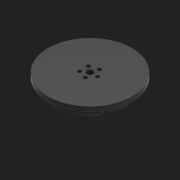
# Autodesk Inventor part: SE02
Saved by Autodesk Inventor 2017 (Build 210142000, 142)
## iProperties
Created: 2019-09-07
Part Number: SE02
Material: ABS Plastic
Document SubType Name: Modeling
Designer: Dell
Density: 1.06 g/cm^3
Appearance: Smooth - Black
Author: Dell
Autodesk Inventor part; units mm, degrees
ref_plane "YZ Plane" through (0, 0, 0) normal (1, 0, 0) x (0, 1, 0)
ref_plane "XZ Plane" through (0, 0, 0) normal (0, 1, 0) x (-1, 0, 0)
ref_plane "XY Plane" through (0, 0, 0) normal (0, 0, 1) x (1, 0, 0)
sketch "Sketch1" plane through (0, 0, 0) normal (0, 0, 1) x (1, 0, 0)
  circle A0 centre (0, 0) radius 15
  circle A1 centre (0, 0) radius 3.5
  dimension "d0" = 30
  dimension "d1" = 7
  constraints: 2 centre point, 2 coincident
  measures "d0" diameter of A0
  measures "d1" diameter of A1
extrude "Extrusion1" add sketch "Sketch1" along normal blind 9
sketch "Sketch2" plane through (0, 0, 9) normal (0, 0, 1) x (1, 0, 0)
  circle A0 centre (0, 0) radius 45
  circle A1 centre (0, 0) radius 3.5 projected
  dimension "d4" = 90
  constraints: 1 centre point, 1 coincident
  measures "d4" diameter of A0
extrude "Extrusion2" add sketch "Sketch2" along normal blind 5
sketch "Sketch14" plane through (0, 0, 9) normal (0, 0, -1) x (-1, 0, 0)
  circle A0 centre (0, 0) radius 18.415 construction
  circle A1 centre (0, 0) radius 3.5 construction
  circle A2 centre (0, 0) radius 15.494 construction
  line L0 (0, 18.415) -> (-38.1, 18.415) construction
  line L1 (-38.1, 18.415) -> (-38.1, 15.494) construction
  line L2 (-38.1, 15.494) -> (0, 15.494) construction
  line L3 (0, 18.415) -> (0, 15.494) construction
  circle A3 centre (0, 0) radius 45 construction
  line L4 (0, 45) -> (0, 19.415)
  circle A4 centre (0, 0) radius 19.415 construction
  line L5 (0, 19.415) -> (-40.5963, 19.415)
  arc A5 (0, 45) -> (-40.5963, 19.415) centre (0, 0) ccw
  line L6 (-12.9177, 14.494) -> (-42.6019, 14.494)
  arc A6 (-12.9177, 14.494) -> (-19.415, 0) centre (0, 0) ccw
  line L7 (-19.415, 0) -> (-45, 0)
  arc A7 (-42.6019, 14.494) -> (-45, 0) centre (0, 0) ccw
  arc A8 (-40.5963, 19.415) -> (-42.6019, 14.494) centre (0, 0) ccw
  line L8 (-39.1, 19.415) -> (-39.1, 14.494)
  dimension "d63" = 36.83
  dimension "d64" = 30.988
  dimension "d65" = 38.1
  dimension "d66" = 1
  dimension "d67" = 1
  dimension "d68" = 1
  dimension "d69" = 1
  constraints: 18 end point, 15 point on circle, 6 horizontal, 5 centre point, 3 coincident, 3 concentric, 3 perpendicular, 3 vertical alignment, 2 point on line, 1 horizontal alignment, 1 vertical, 4 other
  measures "d65" distance of L0.start L0.end
  measures "d67" distance between parallel lines of L5 L0
  measures "d68" distance between parallel lines of L6 L2
  measures "d69" distance between parallel lines of L1 L8
extrude "Extrusion12" add sketch "Sketch14" along normal blind 7 contours L4 L5 A5 | L6 A6 L7 A7
sketch "Sketch15" plane through (0, 0, 9) normal (0, 0, -1) x (-1, 0, 0)
  circle A0 centre (0, 0) radius 39
  arc A1 (-45, 0) -> (0, 45) centre (0, 0) ccw projected
  circle A2 centre (0, 0) radius 45 projected
  dimension "d72" = 78
  constraints: 1 centre point, 1 coincident
  measures "d72" diameter of A0
extrude "Extrusion13" cut sketch "Sketch15" along normal through all
sketch "Sketch16" plane through (0, 0, 0) normal (0, 0, -1) x (-1, 0, 0)
  circle A0 centre (0, 0) radius 11.5
  circle A1 centre (0, 0) radius 3.5 projected
  dimension "d75" = 23
  constraints: 1 centre point, 1 coincident
  measures "d75" diameter of A0
extrude "Extrusion14" add sketch "Sketch16" along normal blind 19
sketch "Sketch17" plane through (0, 0, -19) normal (0, 0, -1) x (-1, 0, 0)
  circle A0 centre (-8, 0) radius 2
  circle A1 centre (0, 0) radius 3.5 construction
  circle A2 centre (0, 0) radius 11.5 construction
  circle A3 centre (-2.4721, -7.6085) radius 2
  circle A4 centre (6.4721, -4.7023) radius 2
  circle A5 centre (6.4721, 4.7023) radius 2
  circle A6 centre (-2.4721, 7.6085) radius 2
  dimension "d78" = 4
  dimension "d79" = 8
  dimension "d82" = 360
  constraints: 5 centre point, 1 horizontal alignment, 11 other
  measures "d78" diameter of A0
  measures "d79" distance of point (0, 0) A0.centre
extrude "Extrusion15" cut sketch "Sketch17" against normal through all
sketch "Sketch19" plane through (0, 0, 0) normal (0, 0, -1) x (-1, 0, 0)
  circle A0 centre (0, 0) radius 11.5 projected
  circle A1 centre (0, 0) radius 15 projected
extrude "Extrusion16" add sketch "Sketch19" along normal blind 1
mirror "Mirror1" about plane through (0, 0, 0) normal (0, 1, 0) remove original yes
sketch "Sketch20" plane through (0, 0, 9) normal (0, 0, -1) x (-1, 0, 0)
  circle A0 centre (0, 0) radius 45 projected
  line L0 (0, -39) -> (0, -19.415) projected
  arc A1 (-33.8239, -19.415) -> (0, -39) centre (0, 0) ccw projected
  line L1 (0, -19.415) -> (-33.8239, -19.415) projected
  circle A2 centre (0, 0) radius 15 projected
  arc A3 (-39, 0) -> (-36.2067, -14.494) centre (0, 0) ccw projected
  line L2 (-19.415, 0) -> (-39, 0) projected
  arc A4 (-19.415, 0) -> (-12.9177, -14.494) centre (0, 0) ccw projected
  line L3 (-36.2067, -14.494) -> (-12.9177, -14.494) projected
  circle A5 centre (0, 0) radius 40
  dimension "d89" = 5
  constraints: 1 centre point
  measures "d89" radial gap between concentric circles of A0 A5
extrude "Extrusion17" cut sketch "Sketch20" against normal blind 2 contours A5
body "Solid1"
